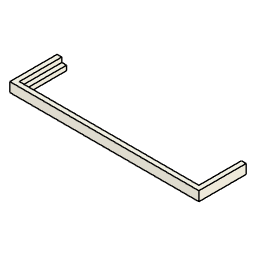
Label Holder (Autodesk Fusion 360 design; units mm, degrees)
Autodesk Fusion 360 part; units mm, degrees
note: some values were not read from the file. Chosen so that the rebuilt part matches the saved one: a side.
sketch "Sketch1" plane through (0, 0, 0) normal (0, 0, 1) x (1, 0, 0)
  line L0 (0, 0) -> (40, 0)
  line L1 (40, 0) -> (40, 10)
  line L2 (0, 0) -> (0, 10)
  line L3 (0, 10) -> (2, 10)
  line L4 (2, 10) -> (2, 2)
  line L5 (2, 2) -> (38, 2)
  line L6 (38, 2) -> (38, 10)
  line L7 (38, 10) -> (40, 10)
  dimension "d1" = 40
  dimension "d2" = 2
  dimension "d3" = 2
  dimension "d4" = 10
  constraint coincident L0.start L2.start
  constraint horizontal L0
  constraint perpendicular L0 L1
  constraint perpendicular L0 L2
  constraint perpendicular L2 L3
  constraint perpendicular L0 L4
  constraint perpendicular L4 L5
  constraint perpendicular L5 L6
  constraint perpendicular L1 L7
  constraint equal L3 L7
  measures "d1" distance of L0.start L0.end
  measures "d2" distance of L2.end L3.end
  measures "d3" distance of L0 L5
  measures "d4" distance of L0.start L2.end
extrude "Extrude1" add sketch "Sketch1" along normal blind 1 thin wall 1 on the left open curves L1 L0 L2
extrude "Extrude2" add sketch "Sketch1" against normal blind 1
equation "d3 = d2"
